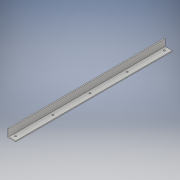
# Autodesk Inventor part: Bumper L
Saved by Autodesk Inventor 2018 (Build 220112000, 112)
## iProperties
Created: 2019-02-24
Part Number: Bumper L
Material: Generic
Document SubType Name: Modeling
Designer: maste
Density: 1 g/cm^3
Appearance: Default
Author: maste
Autodesk Inventor part; units mm, degrees
ref_plane "YZ Plane" through (0, 0, 0) normal (1, 0, 0) x (0, 1, 0)
ref_plane "XZ Plane" through (0, 0, 0) normal (0, 1, 0) x (-1, 0, 0)
ref_plane "XY Plane" through (0, 0, 0) normal (0, 0, 1) x (1, 0, 0)
sketch "Sketch1" plane through (0, 0, 0) normal (0, 0, 1) x (1, 0, 0)
  line L0 (0, 0) -> (3.175, 0)
  line L1 (3.175, 0) -> (3.175, 25.4)
  line L2 (3.175, 25.4) -> (0, 25.4)
  line L3 (0, 25.4) -> (0, 0)
  line L4 (0, 0) -> (25.4, 0)
  line L5 (25.4, 0) -> (25.4, 3.175)
  line L6 (25.4, 3.175) -> (0, 3.175)
  line L7 (0, 3.175) -> (0, 0)
  dimension "d0" = 3.175
  dimension "d1" = 25.4
  dimension "d2" = 25.4
  dimension "d3" = 3.175
  constraints: 16 end point, 4 parallel, 2 horizontal, 2 perpendicular
  measures "d0" distance of L2.end L1.end
  measures "d1" distance of L1.end L0.end
  measures "d2" distance of L6.end L5.end
  measures "d3" distance of L5.end L4.end
extrude "Extrusion1" add sketch "Sketch1" along normal blind 508
sketch "Sketch2" plane through (3.175, 3.175, 0) normal (0, 1, 0) x (1, 0, 0)
  line L0 (-3.175, 0) -> (9.525, 0) construction
  line L1 (22.225, 0) -> (0, 0) construction
  line L2 (9.525, 0) -> (9.525, -12.7) construction
  circle A0 centre (9.525, -12.7) radius 2.5797
  line L3 (-3.175, -508) -> (22.225, -508) construction
  line L4 (9.525, -508) -> (9.525, -495.3) construction
  circle A1 centre (9.525, -495.3) radius 2.5826
  line L5 (-3.175, 0) -> (-3.175, -508) construction
  line L6 (-3.175, -254) -> (22.225, -254) construction
  line L7 (22.225, 0) -> (22.225, -508) construction
  line L8 (9.525, -495.3) -> (9.525, -254) construction
  circle A2 centre (9.525, -374.65) radius 2.5826
  circle A3 centre (9.525, -254) radius 2.5826
  line L9 (9.525, -254) -> (9.525, -12.7) construction
  circle A4 centre (9.525, -133.35) radius 2.5826
  dimension "d6" = 12.7
  dimension "d7" = 12.7
  dimension "d16" = 12.7
  constraints: 12 end point, 6 midpoint, 5 centre point, 3 coincident, 1 perpendicular, 1 point on line, 1 vertical
  measures "d6" distance of L0.start L0.end
  measures "d7" distance of L0.end L2.end
  measures "d16" distance of L4.start L4.end
extrude "Extrusion3" cut sketch "Sketch2" against normal blind 533.4
body "Solid1"
